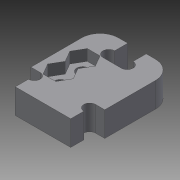
# Autodesk Inventor part: Carriage_Joint_Boltblock
Saved by Autodesk Inventor 2014 (Build 180170000, 170)
## iProperties
Created: 2014-11-10
Part Number: Carriage_Joint_Boltblock
Material: Generic
Document SubType Name: Modeling
Designer: ThatOtherGuy
Density: 1 g/cm^3
Appearance: Default
Author: ThatOtherGuy
Autodesk Inventor part; units mm, degrees
ref_plane "YZ Plane" through (0, 0, 0) normal (1, 0, 0) x (0, 1, 0)
ref_plane "XZ Plane" through (0, 0, 0) normal (0, 1, 0) x (-1, 0, 0)
ref_plane "XY Plane" through (0, 0, 0) normal (0, 0, 1) x (1, 0, 0)
sketch "Sketch1" plane through (0, 0, 0) normal (0, 0, 1) x (1, 0, 0)
  line L0 (0, 0) -> (2.5, 0)
  line L1 (2.5, 0) -> (2.5, -6.731)
  line L2 (2.5, -6.731) -> (17.5, -6.731)
  line L3 (17.5, -6.731) -> (17.5, 0)
  line L4 (17.5, 0) -> (20, 0)
  line L5 (20, 0) -> (20, 18.731)
  line L6 (20, 18.731) -> (12.5, 18.731)
  line L7 (12.5, 18.731) -> (12.5, 12)
  line L8 (12.5, 12) -> (7.5, 12)
  line L9 (7.5, 12) -> (7.5, 18.731)
  line L10 (7.5, 18.731) -> (0, 18.731)
  line L11 (0, 18.731) -> (0, 0)
  dimension "d0" = 15
  dimension "d1" = 20
  dimension "d3" = 6.731
  dimension "d4" = 5
  dimension "d5" = 12
  constraints: 24 end point, 9 parallel, 5 equal length, 1 collinear, 1 horizontal, 1 perpendicular
  measures "d0" distance of L1.end L2.end
  measures "d1" distance between parallel lines of L5 L11
  measures "d3" distance of L6.end L7.end
  measures "d4" distance of L7.end L8.end
  measures "d5" distance between parallel lines of L4 L8
extrude "Extrusion1" add sketch "Sketch1" along normal blind 6.731
sketch "Sketch2" plane through (0, 0, 0) normal (0, 0, -1) x (-1, 0, 0)
  line L0 (0, 0) -> (-2.5, 0) projected
  circle A0 centre (-5, 3) radius 1.588
  circle A1 centre (-5, 9) radius 1.588
  line L1 (-12.5, 12) -> (-7.5, 12) projected
  line L2 (-2.5, 0) -> (-2.5, -6.731) projected
  line L3 (-10, 12) -> (-10, 9.3655) construction
  dimension "d8" = 6
  dimension "d9" = 3.176
  dimension "d10" = 3
  dimension "d22" = 5
  constraints: 2 centre point, 2 end point, 1 equal radius, 1 midpoint, 1 parallel, 1 vertical alignment
  measures "d8" distance of A0.centre A1.centre
  measures "d9" diameter of A1
  measures "d10" distance from line of L0 A0.centre
  measures "d22" distance from line of L3 A1.centre
extrude "Extrusion2" cut sketch "Sketch2" against normal up to next
fillet "Fillet1" radius 5 2 edges at (0, 18.731, 3.3655) (20, 18.731, 3.3655)
sketch "Sketch3" plane through (0, 0, 6.731) normal (0, 0, 1) x (1, 0, 0)
  circle A0 centre (5, 3) radius 1.588 projected
  circle A1 centre (5, 9) radius 1.588 projected
  line L0 (8.4641, 9) -> (6.7321, 6)
  line L1 (6.7321, 6) -> (3.2679, 6)
  line L2 (3.2679, 6) -> (1.5359, 9)
  line L3 (1.5359, 9) -> (3.2679, 12)
  line L4 (3.2679, 12) -> (6.7321, 12)
  line L5 (6.7321, 12) -> (8.4641, 9)
  line L6 (8.4641, 3) -> (6.7321, 0)
  line L7 (6.7321, 0) -> (3.2679, 0)
  line L8 (3.2679, 0) -> (1.5359, 3)
  line L9 (1.5359, 3) -> (3.2679, 6)
  line L10 (3.2679, 6) -> (6.7321, 6)
  line L11 (6.7321, 6) -> (8.4641, 3)
  dimension "d14" = 6
  constraints: 24 end point, 2 coincident, 2 horizontal, 1 collinear, 26 other
  measures "d14" distance between parallel lines of L4 L1
extrude "Extrusion3" cut sketch "Sketch3" against normal blind 3
sketch "Sketch4" plane through (0, 0, 6.731) normal (0, 0, 1) x (1, 0, 0)
  circle A0 centre (7.5, 13.5875) radius 1.5875
  circle A1 centre (12.5, 13.5875) radius 1.5875
  line L0 (12.5, 18.731) -> (12.5, 12) projected
  line L1 (0, 0) -> (2.5, 0) projected
  line L2 (2.5, 0) -> (2.5, -6.731) projected
  line L3 (17.5, -6.731) -> (17.5, 0) projected
  line L4 (17.5, 0) -> (20, 0) projected
  arc A2 (2.5, -3.175) -> (2.5, 0) centre (2.5, -1.5875) ccw
  arc A3 (17.5, 0) -> (17.5, -3.175) centre (17.5, -1.5875) ccw
  dimension "d17" = 3.175
  constraints: 4 point on circle, 3 centre point, 3 point on line, 2 equal radius, 2 tangent, 1 horizontal alignment, 1 vertical alignment, 3 other
  measures "d17" diameter of A0
extrude "Extrusion4" cut sketch "Sketch4" against normal up to next
equation "\"d3\" = THICKB"
equation "\"d6\" = THICKB"
equation "\"THICKA\" = 3.175"
equation "\"THICKB\" = 6.731"
equation "\"THICKC\" = 12.7"
equation "\"THICKPLY\" = 5"
equation "\"MAGDIA\" = 9.5"
equation "\"BALLDIA\" = 12"
body "Solid1"
